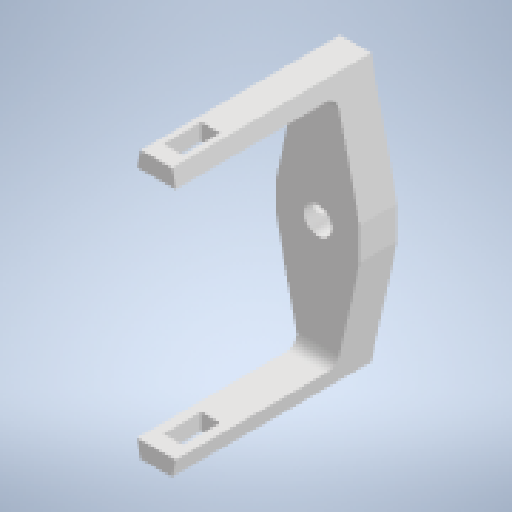
# Autodesk Inventor part: TurretPressFit
Saved by Autodesk Inventor 2023 (Build 270158000, 158)
## iProperties
Created: 2023-05-07
Part Number: TurretPressFit
Material: Generic
Document SubType Name: Modeling
Designer: karpova
Density: 1 g/cm^3
Appearance: Default
Author: karpova
Autodesk Inventor part; units mm, degrees
ref_plane "YZ Plane" through (0, 0, 0) normal (1, 0, 0) x (0, 1, 0)
ref_plane "XZ Plane" through (0, 0, 0) normal (0, 1, 0) x (-1, 0, 0)
ref_plane "XY Plane" through (0, 0, 0) normal (0, 0, 1) x (1, 0, 0)
sketch "Sketch1" plane through (0, 0, 0) normal (0, 0, 1) x (1, 0, 0)
  arc A0 (-9.2513, -12.8456) -> (-7.7191, -13.7193) centre (-8.2517, -12.873) ccw projected
  line L0 (-7.7191, -13.7193) -> (-1.0653, -9.532) projected
  arc A1 (1.0653, -9.532) -> (-1.0653, -9.532) centre (0, -11.2247) ccw projected
  line L1 (1.0653, -9.532) -> (7.7191, -13.7193) projected
  arc A2 (7.7191, -13.7193) -> (9.2513, -12.8456) centre (8.2517, -12.873) ccw projected
  arc A3 (12.8456, -9.2513) -> (9.2513, -12.8456) centre (12.75, -12.75) ccw projected
  arc A4 (12.8456, -9.2513) -> (13.7193, -7.7191) centre (12.873, -8.2517) ccw projected
  line L2 (13.7193, -7.7191) -> (9.532, -1.0653) projected
  arc A5 (9.532, 1.0653) -> (9.532, -1.0653) centre (11.2247, 0) ccw projected
  line L3 (9.532, 1.0653) -> (13.7385, 7.7495) projected
  line L4 (7.7677, 13.7499) -> (1.0653, 9.532) projected
  arc A6 (-1.0653, 9.532) -> (1.0653, 9.532) centre (0, 11.2247) ccw projected
  line L5 (-1.0653, 9.532) -> (-7.7191, 13.7193) projected
  arc A7 (-7.7191, 13.7193) -> (-9.2513, 12.8456) centre (-8.2517, 12.873) ccw projected
  arc A8 (-12.8456, 9.2513) -> (-9.2513, 12.8456) centre (-12.75, 12.75) ccw projected
  arc A9 (-12.8456, 9.2513) -> (-13.7193, 7.7191) centre (-12.873, 8.2517) ccw projected
  line L6 (-13.7193, 7.7191) -> (-9.532, 1.0653) projected
  arc A10 (-9.532, -1.0653) -> (-9.532, 1.0653) centre (-11.2247, 0) ccw projected
  line L7 (-9.532, -1.0653) -> (-13.7193, -7.7191) projected
  arc A11 (-13.7193, -7.7191) -> (-12.8456, -9.2513) centre (-12.873, -8.2517) ccw projected
  arc A12 (-9.2513, -12.8456) -> (-12.8456, -9.2513) centre (-12.75, -12.75) ccw projected
  circle A13 centre (0, 0) radius 2.5 projected
  circle A14 centre (0, 0) radius 2 projected
  circle A15 centre (0, 0) radius 2.1
  line L8 (2.8, -24.1) -> (-2.8, -24.1)
  line L9 (-2.8, 24.1) -> (2.8, 24.1)
  line L10 (2.8, -24.1) -> (7.5, -2.9)
  line L11 (7.5, 2.9) -> (2.8, 24.1)
  line L12 (-2.8, 24.1) -> (-7.5, 2.9)
  line L13 (-7.5, -2.9) -> (-2.8, -24.1)
  line L14 (7.5, -2.9) -> (7.5, 2.9)
  line L15 (-7.5, 2.9) -> (-7.5, -2.9)
  line L16 (7.5, -2.9) -> (-7.5, -2.9) construction
  line L17 (-7.5, 2.9) -> (7.5, 2.9) construction
  line L18 (2.8, -24.1) -> (2.8, 24.1) construction
  line L19 (-2.8, 24.1) -> (-2.8, -24.1) construction
  line L20 (7.5, 0) -> (0, 0) construction
  line L21 (0, 0) -> (-7.5, 0) construction
  line L22 (-2.5, -2.9) -> (-2.5, 2.9) construction
  arc A16 (9.3, 12.8764) -> (7.7677, 13.7499) centre (8.3003, 12.9036) ccw projected
  arc A17 (13.7385, 7.7495) -> (12.8714, 9.2819) centre (12.8922, 8.2822) ccw projected
  arc A18 (9.3, 12.8764) -> (12.8714, 9.2819) centre (12.7987, 12.7812) ccw projected
  dimension "d0" = 0.1
  dimension "d5" = 48.2
  dimension "d6" = 5.6
  dimension "d7" = 5
  dimension "d8" = 5.8
  constraints: 30 end point, 4 horizontal, 4 parallel, 3 vertical, 2 coincident, 2 midpoint, 2 point on line, 1 centre point, 1 collinear, 1 perpendicular, 1 tangent
  measures "d0" radial gap between concentric circles of A15 A14
  measures "d5" distance between parallel lines of L8 L9
  measures "d6" distance of L9.start L9.end
  measures "d7" distance between parallel lines of L15 L22
  measures "d8" distance of L12.end L13.start
extrude "Extrusion1" add sketch "Sketch1" along normal blind 6.8 contours L13 L15 L12 L5 A6 L4 L11 L14 L10 L1 A1 L0 | L0 A1 L1 L10 L8 L13 | L12 L9 L11 L4 A6 L5
sketch "Sketch2" plane through (-7.5, -2.9, 0) normal (-1, 0, 0) x (0, 0, 1)
  line L0 (0, 5.8) -> (0, 0) projected
  line L1 (0, 0) -> (6.8, 0) projected
  line L2 (6.8, 5.8) -> (6.8, 0) projected
  line L3 (0, 5.8) -> (6.8, 5.8) projected
  circle A0 centre (3.4, 2.9) radius 1.6
  point P0 (0, 2.9)
  dimension "d9" = 3.2
  constraints: 1 centre point
  measures "d9" diameter of A0
extrude "Extrusion2" cut sketch "Sketch2" against normal blind 7.4875 contours A0
sketch "Sketch3" plane through (0, 0, 6.8) normal (0, 0, 1) x (1, 0, 0)
  line L0 (7.5, 2.9) -> (2.8, 24.1) projected
  line L1 (2.8, 24.1) -> (-2.8, 24.1) projected
  line L2 (-2.8, 24.1) -> (-7.5, 2.9) projected
  line L3 (-7.5, 2.9) -> (-7.5, -2.9) projected
  line L4 (-7.5, -2.9) -> (-2.8, -24.1) projected
  line L5 (-2.8, -24.1) -> (2.8, -24.1) projected
  line L6 (2.8, -24.1) -> (7.5, -2.9) projected
  line L7 (7.5, -2.9) -> (7.5, 2.9) projected
  circle A0 centre (0, 0) radius 2.5 projected
  line L8 (3.4651, -21.1) -> (-3.4651, -21.1)
  line L9 (-3.4651, 21.1) -> (3.4651, 21.1)
  point P0 (0, 0)
  dimension "d19" = 3
  dimension "d20" = 3
  constraints: 4 end point, 4 point on line, 1 horizontal, 1 parallel
  measures "d19" distance between parallel lines of L1 L9
  measures "d20" distance between parallel lines of L5 L8
extrude "Extrusion3" add sketch "Sketch3" along normal blind 29.1 contours L9 L2 L1 L0 | L6 L5 L4 L8
sketch "Sketch4" plane through (-2.8, 24.1, 0) normal (0, 1, 0) x (1, 0, 0)
  line L0 (5.6, 0) -> (0, 0) construction
  line L1 (0, 0) -> (0, -35.9) construction
  line L2 (5.6, 0) -> (5.6, -35.9) construction
  line L3 (5.6, -35.9) -> (0, -35.9) projected
  line L4 (6.2651, -35.9) -> (-0.6651, -35.9) construction
  line L5 (2.8, -35.9) -> (2.8, 0) construction
  line L6 (5.6, -32.9) -> (0, -32.9) construction
  line L7 (4.5, -32.9) -> (1.1, -32.9)
  line L8 (1.1, -32.9) -> (1.1, -26.1)
  line L9 (1.1, -26.1) -> (4.5, -26.1)
  line L10 (4.5, -26.1) -> (4.5, -32.9)
  dimension "d23" = 3
  dimension "d25" = 3.4
  dimension "d26" = 6.8
  constraints: 12 end point, 3 point on line, 2 parallel, 2 perpendicular, 1 horizontal, 1 midpoint, 1 vertical, 1 other
  measures "d23" distance between parallel lines of L3 L6
  measures "d25" distance of L8.end L9.end
  measures "d26" distance of L7.end L8.end
extrude "Extrusion4" cut sketch "Sketch4" against normal through all
fillet "Fillet1" radius 2 2 edges at (0, -21.1, 6.8) (0, 21.1, 6.8)
equation "\"d20\" = d19"
equation "\"d26\" = 2 * d25"
body "Solid1"
